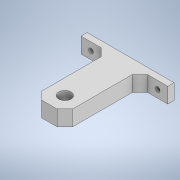
# Autodesk Inventor part: suporte barra
Saved by Autodesk Inventor 2022 (Build 260153000, 153)
## iProperties
Created: 2022-02-16
Part Number: suporte barra
Material: Genérico
Document SubType Name: Modeling
Designer: mathe
Density: 1 g/cm^3
Appearance: Padrão
Author: mathe
Autodesk Inventor part; units mm, degrees
ref_plane "YZ Plane" through (0, 0, 0) normal (1, 0, 0) x (0, 1, 0)
ref_plane "XZ Plane" through (0, 0, 0) normal (0, 1, 0) x (-1, 0, 0)
ref_plane "XY Plane" through (0, 0, 0) normal (0, 0, 1) x (1, 0, 0)
sketch "Esboço1" plane through (0, 0, 0) normal (0, 0, 1) x (1, 0, 0)
  line L0 (0, 0) -> (56, 0)
  line L1 (56, 0) -> (56, 10)
  line L2 (56, 10) -> (0, 10)
  line L3 (0, 10) -> (0, 0)
  line L4 (18, 10) -> (38, 10)
  line L5 (38, 10) -> (38, 0)
  line L6 (38, 0) -> (18, 0)
  line L7 (18, 0) -> (18, 10)
  line L8 (18, 10) -> (38, 0) construction
  line L9 (38, 10) -> (18, 0) construction
  point P0 (28, 5)
  dimension "d0" = 56
  dimension "d1" = 10
  dimension "d2" = 20
  constraints: 20 end point, 4 parallel, 2 horizontal, 2 midpoint, 2 perpendicular, 1 point on line
  measures "d0" distance of L2.end L1.end
  measures "d1" distance of L1.end L0.end
  measures "d2" distance of L5.end L6.end
extrude "Extrusão1" add sketch "Esboço1" along normal blind 4 contours L3 L2 L7 L0 | L5 L2 L1 L0
extrude "Extrusão2" add sketch "Esboço1" along normal blind 52.426 contours L7 L2 L5 L0
chamfer "Chanfro1" distance 5 angle 45 4 edges at (38, 5, 4) (18, 5, 4) (38, 5, 52.426) (18, 5, 52.426)
sketch "Esboço2" plane through (0, 10, 0) normal (0, 1, 0) x (1, 0, 0)
  line L0 (33, -52.426) -> (23, -52.426) projected
  point P0 (0, 0)
  point P1 (28, -42.426)
  dimension "d24" = 10
  measures "d24" distance from line of L0 point (28, -42.426)
hole "Furo1" at (28, 10, 42.426) direction (0, -1, 0) diameter 8 end through all
sketch "Esboço3" plane through (0, 0, 4) normal (0, 0, 1) x (1, 0, 0)
  point P0 (0, 0)
  point P1 (6.5, 5)
  point P2 (49.5, 5)
hole "Furo2" at (6.5, 5, 4) at (49.5, 5, 4) direction (0, 0, -1) diameter 3 end through all
